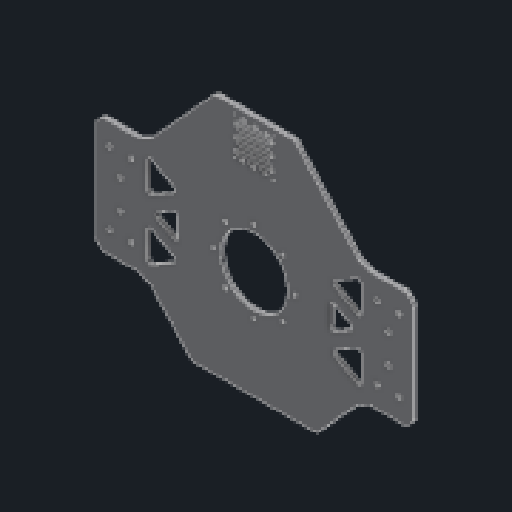
# Autodesk Inventor part: Root
Saved by Autodesk Inventor 2025.2 (Build 292293000, 293)
## iProperties
Created: 2020-05-07
Part Number: Root
Material: Generic
Document SubType Name: Sheet Metal
Designer: valer
Density: 1 g/cm^3
Sheet Metal Rule: Default
Appearance: Default
Author: valer
Autodesk Inventor part; units mm, degrees
ref_plane "YZ Plane" through (0, 0, 0) normal (1, 0, 0) x (0, 1, 0)
ref_plane "XZ Plane" through (0, 0, 0) normal (0, 1, 0) x (-1, 0, 0)
ref_plane "XY Plane" through (0, 0, 0) normal (0, 0, 1) x (1, 0, 0)
sketch "Base" plane through (0, 0, 0) normal (0, 0, 1) x (1, 0, 0)
  circle A0 centre (-56.25, 0) radius 2.75 construction
  circle A1 centre (0, -56.25) radius 2.75 construction
  circle A2 centre (0, 56.25) radius 2.75 construction
  circle A3 centre (39.7748, -39.7748) radius 2.75 construction
  circle A4 centre (-39.7748, 39.7748) radius 2.75 construction
  circle A5 centre (-39.7748, -39.7748) radius 2.75 construction
  circle A6 centre (39.7748, 39.7748) radius 2.75 construction
  circle A7 centre (56.25, 0) radius 2.75 construction
  circle A8 centre (0, 0) radius 45 construction
  circle A9 centre (0, 0) radius 61
  line L0 (220, 80) -> (-220, 80) construction
  line L1 (0, -210) -> (0, 210) construction
  line L2 (-308, 0) -> (308, 0) construction
  line L3 (-220, 80) -> (-150, 80)
  line L4 (-150, 80) -> (-150, 0)
  line L5 (-150, 0) -> (-220, 0)
  line L6 (-220, 0) -> (-220, 80)
  line L7 (86.6025, -150) -> (-86.6025, -150)
  line L8 (-86.6025, -150) -> (-173.2051, 0)
  line L9 (-173.2051, 0) -> (-86.6025, 150)
  line L10 (-86.6025, 150) -> (86.6025, 150)
  line L11 (86.6025, 150) -> (173.2051, 0)
  line L12 (173.2051, 0) -> (86.6025, -150)
  line L13 (-150, 0) -> (-86.6025, 150) construction
  line L14 (220, 80) -> (150, 80)
  line L15 (150, 80) -> (150, 0)
  line L16 (150, 0) -> (220, 0)
  line L17 (220, 0) -> (220, 80)
  line L18 (150, 0) -> (86.6025, 150) construction
  line L19 (-220, -80) -> (-150, -80)
  line L20 (-150, -80) -> (-150, 0)
  line L21 (-150, 0) -> (-219.7895, 0)
  line L22 (-219.7895, 0) -> (-220, -80)
  line L23 (-150, 0) -> (-86.6025, -150) construction
  line L24 (220, 0) -> (220, -80)
  line L25 (220, -80) -> (150, -80)
  line L26 (150, -80) -> (150, 0)
  line L27 (150, 0) -> (220, 0)
  line L28 (150, 0) -> (86.6025, -150) construction
  circle A10 centre (0, 0) radius 46.5
  circle A11 centre (-56.25, 0) radius 2.25
  circle A12 centre (-39.7748, -39.7748) radius 2.25
  circle A13 centre (0, -56.25) radius 2.25
  circle A14 centre (39.7748, -39.7748) radius 2.25
  circle A15 centre (56.25, 0) radius 2.25
  circle A16 centre (39.7748, 39.7748) radius 2.25
  circle A17 centre (0, 56.25) radius 2.25
  circle A18 centre (-39.7748, 39.7748) radius 2.25
  line L29 (-150, 80) -> (-86.6025, 150)
  line L30 (86.6025, 150) -> (150, 80)
  line L31 (-150, -80) -> (-86.6025, -150)
  line L32 (86.6025, -150) -> (150, -80)
  point P0 (0, 0)
  point P1 (210, 0)
  point P2 (150, 40.1924)
  point P3 (150, -40.1924)
  point P4 (173.2051, 0)
  point P5 (173.2051, 0)
  point P6 (-150, 40.1924)
  point P7 (-173.2051, 0)
  point P8 (-173.2051, 0)
  point P9 (-150, -40.1924)
  point P10 (173.2051, 0)
  point P11 (-173.2051, 0)
  point P12 (-173.2051, 0)
  dimension "d89" = 80
  dimension "d90" = 70
  dimension "d91" = 1.5
  dimension "d92" = 4.5
  dimension "d157" = 150
  dimension "d158" = 220
  measures "d89" distance between parallel lines of L0 L5
  measures "d90" distance between parallel lines of L4 L6
  measures "d91" radial gap between concentric circles of A10 A8
  measures "d92" diameter of A11
  measures "d157" distance from line of L7 A8.centre
  measures "d158" distance between parallel lines of L24 L1
extrude "Plate1" add sketch "Base" against normal blind 5 contours A9 | L3 L4 L9 L5 L6 | L29 L9 L4 | L9 L10 L11 L15 L26 L12 L7 L8 L20 L4 | L4 L5 L9 | L5 L8 L20 L19 L22 | L20 L8 L5 | L30 L15 L11 | L8 L31 L20 | L15 L14 L17 L16 L11 | L11 L16 L15 | L16 L24 L25 L26 L12 | L12 L26 L16 | L12 L26 L32
sketch "LegMountHoles" plane through (0, 0, -5) normal (0, 0, -1) x (-1, 0, 0)
  line L0 (-222.4542, 0) -> (-220, 0) construction
  line L1 (-220, 80) -> (-150, 80) construction
  line L2 (-185, 80) -> (-185, 0) construction
  line L3 (-170, 58) -> (-200, 58) construction
  circle A0 centre (-170, 58) radius 3
  circle A1 centre (-200, 58) radius 3
  circle A2 centre (-185, 18) radius 3
  line L4 (308.4908, 0) -> (-310.9451, 0) construction
  line L5 (0, -210) -> (0, 210) construction
  circle A3 centre (170, 58) radius 3
  circle A4 centre (200, 58) radius 3
  circle A5 centre (185, 18) radius 3
  circle A6 centre (-170, -58) radius 3
  circle A7 centre (-200, -58) radius 3
  circle A8 centre (-185, -18) radius 3
  circle A9 centre (170, -58) radius 3
  circle A10 centre (200, -58) radius 3
  circle A11 centre (185, -18) radius 3
  line L6 (-150, 80) -> (-86.6025, 150) projected
  line L7 (-220, -80) -> (-220, 80) projected
  point P0 (0, 0)
  point P1 (-185, 58)
  dimension "d93" = 6
  dimension "d94" = 30
  dimension "d95" = 40
  dimension "d161" = 18
  constraints: 12 centre point, 9 symmetric about line, 6 end point, 4 point on line, 2 coincident, 2 equal radius, 2 horizontal, 2 midpoint, 2 perpendicular, 1 collinear, 9 other
  measures "d93" diameter of A0
  measures "d94" distance of L3.start L3.end
  measures "d95" distance from line of L3 A2.centre
  measures "d161" distance from line of L4 A2.centre
extrude "LegMountHolesFeature" cut sketch "LegMountHoles" against normal blind 5
chamfer "OutsideChamfersFeature" distance 10 angle 45 8 edges at (-220, -80, -2.5) (-150, -80, -2.5) (150, -80, -2.5) (220, -80, -2.5) (-220, 80, -2.5) (-150, 80, -2.5) (150, 80, -2.5) (220, 80, -2.5)
fillet "OutsideFilletsFeature" radius 8 18 edges at (160, 80, -2.5) (210, 80, -2.5) (220, 70, -2.5) (210, -80, -2.5) (160, -80, -2.5) (86.6025, -150, -2.5) (-86.6025, -150, -2.5) (-160, -80, -2.5) (-210, -80, -2.5) (-219.9737, -70, -2.5) (-220, 0, -2.5) (-220, 70, -2.5) (-210, 80, -2.5) (-160, 80, -2.5) (-143.2871, 87.412, -2.5) (143.2871, 87.412, -2.5) (143.2871, -87.412, -2.5) (-143.2871, -87.412, -2.5)
sketch "LaserMount" plane through (0, 0, -5) normal (0, 0, -1) x (-1, 0, 0)
  line L0 (86.6025, 150) -> (142.1497, 88.6679)
  line L1 (86.6025, 150) -> (54.9038, 185)
  line L2 (54.9038, 185) -> (0, 185)
  line L3 (0, -217) -> (0, 252) construction
  line L4 (-86.6025, 150) -> (86.6025, 150)
  line L5 (-86.6025, 150) -> (-54.9038, 185)
  line L6 (-54.9038, 185) -> (0, 185)
  line L7 (86.6025, 150) -> (142.1497, 88.6679)
  point P0 (0, 0)
  dimension "d119" = 35
  measures "d119" distance between parallel lines of L2 L4
sheet face with bend "LaserMountFeature" sketch "LaserMount" thickness 5 toward (0, 0, 1) bend radius 5 relief straight relief width 5 relief depth 2.5
bend "Bend4"
fillet "FrontFilletsFeature" radius 8 2 edges at (-54.9038, 185, -2.5) (54.9038, 185, -2.5)
sketch "Sketch13" plane through (0, 0, -5) normal (0, 0, -1) x (-1, 0, 0)
  circle A0 centre (26.5, 175.5) radius 1
  circle A1 centre (26.5, 122.5) radius 1
  circle A2 centre (-26.5, 122.5) radius 1
  circle A3 centre (-26.5, 175.5) radius 1
  circle A4 centre (-26.5, 175.5) radius 1.5
  circle A5 centre (-26.5, 122.5) radius 1.5 construction
  arc A6 (26, 119.25) -> (29.75, 123) centre (26, 123) ccw construction
  line L0 (26, 119.25) -> (-26, 119.25) construction
  arc A7 (-29.75, 123) -> (-26, 119.25) centre (-26, 123) ccw construction
  line L1 (-29.75, 123) -> (-29.75, 175) construction
  arc A8 (-26, 178.75) -> (-29.75, 175) centre (-26, 175) ccw construction
  line L2 (-26, 178.75) -> (26, 178.75) construction
  arc A9 (29.75, 175) -> (26, 178.75) centre (26, 175) ccw construction
  line L3 (29.75, 175) -> (29.75, 123) construction
  circle A10 centre (26.5, 122.5) radius 1.5 construction
  circle A11 centre (-26.5, 175.5) radius 1.5 construction
  circle A12 centre (26.5, 175.5) radius 1.5
  circle A13 centre (-26.5, 122.5) radius 1.5 construction
  spline S0 degree 3 poles (23.6196, 120.808) (23.6757, 120.7125) (23.7146, 120.6074) (23.7573, 120.3902) (23.7611, 120.278) (23.7347, 120.0723) (23.7049, 119.9435) (23.5614, 119.6936) (23.4754, 119.5942) (23.2857, 119.4454) (23.1885, 119.3933) (22.9792, 119.3212) (22.8686, 119.3024) (22.7579, 119.3024) knots 0 0 0 0 0.207802 0.207802 0.415412 0.415412 0.597058 0.597058 0.743635 0.743635 0.871765 0.871765 1 1 1 1 construction
  arc A14 (28.192, 125.3804) -> (23.6196, 120.808) centre (26.5, 122.5) ccw construction
  spline S1 degree 3 poles (29.6976, 126.2421) (29.6976, 126.1314) (29.6779, 126.0211) (29.6047, 125.8121) (29.5512, 125.7135) (29.4244, 125.5497) (29.3335, 125.4537) (29.083, 125.3108) (28.9586, 125.2686) (28.7195, 125.2364) (28.6093, 125.2407) (28.3924, 125.2846) (28.2875, 125.3243) (28.192, 125.3804) knots 0 0 0 0 0.208148 0.208148 0.416054 0.416054 0.597577 0.597577 0.743842 0.743842 0.871851 0.871851 1 1 1 1 construction
  line L4 (29.6976, 171.7579) -> (29.6976, 126.2421) construction
  spline S2 degree 3 poles (28.192, 172.6196) (28.2875, 172.6757) (28.3926, 172.7146) (28.6098, 172.7573) (28.722, 172.7611) (28.9277, 172.7347) (29.0565, 172.7049) (29.3064, 172.5614) (29.4058, 172.4754) (29.5546, 172.2857) (29.6067, 172.1885) (29.6788, 171.9792) (29.6976, 171.8686) (29.6976, 171.7579) knots 0 0 0 0 0.207802 0.207802 0.415412 0.415412 0.597058 0.597058 0.743635 0.743635 0.871765 0.871765 1 1 1 1 construction
  arc A15 (23.6196, 177.192) -> (28.192, 172.6196) centre (26.5, 175.5) ccw construction
  spline S3 degree 3 poles (22.7579, 178.6976) (22.8686, 178.6976) (22.9789, 178.6779) (23.1879, 178.6047) (23.2865, 178.5512) (23.4503, 178.4244) (23.5463, 178.3335) (23.6892, 178.083) (23.7314, 177.9586) (23.7636, 177.7195) (23.7593, 177.6093) (23.7154, 177.3924) (23.6757, 177.2875) (23.6196, 177.192) knots 0 0 0 0 0.208148 0.208148 0.416054 0.416054 0.597577 0.597577 0.743842 0.743842 0.871851 0.871851 1 1 1 1 construction
  line L5 (-22.7579, 178.6976) -> (22.7579, 178.6976) construction
  spline S4 degree 3 poles (-23.6196, 177.192) (-23.6757, 177.2875) (-23.7146, 177.3926) (-23.7573, 177.6098) (-23.7611, 177.722) (-23.7347, 177.9277) (-23.7049, 178.0565) (-23.5614, 178.3064) (-23.4754, 178.4058) (-23.2857, 178.5546) (-23.1885, 178.6067) (-22.9792, 178.6788) (-22.8686, 178.6976) (-22.7579, 178.6976) knots 0 0 0 0 0.207802 0.207802 0.415412 0.415412 0.597058 0.597058 0.743635 0.743635 0.871765 0.871765 1 1 1 1 construction
  arc A16 (-28.192, 172.6196) -> (-23.6196, 177.192) centre (-26.5, 175.5) ccw construction
  spline S5 degree 3 poles (-29.6976, 171.7579) (-29.6976, 171.8686) (-29.6779, 171.9789) (-29.6047, 172.1879) (-29.5512, 172.2865) (-29.4244, 172.4503) (-29.3335, 172.5463) (-29.083, 172.6892) (-28.9586, 172.7314) (-28.7195, 172.7636) (-28.6093, 172.7593) (-28.3924, 172.7154) (-28.2875, 172.6757) (-28.192, 172.6196) knots 0 0 0 0 0.208148 0.208148 0.416054 0.416054 0.597577 0.597577 0.743842 0.743842 0.871851 0.871851 1 1 1 1 construction
  line L6 (-29.6976, 126.2421) -> (-29.6976, 171.7579) construction
  spline S6 degree 3 poles (-28.192, 125.3804) (-28.2875, 125.3243) (-28.3926, 125.2854) (-28.6098, 125.2427) (-28.722, 125.2389) (-28.9277, 125.2653) (-29.0565, 125.2951) (-29.3064, 125.4386) (-29.4058, 125.5246) (-29.5546, 125.7143) (-29.6067, 125.8115) (-29.6788, 126.0208) (-29.6976, 126.1314) (-29.6976, 126.2421) knots 0 0 0 0 0.207802 0.207802 0.415412 0.415412 0.597058 0.597058 0.743635 0.743635 0.871765 0.871765 1 1 1 1 construction
  arc A17 (-23.6196, 120.808) -> (-28.192, 125.3804) centre (-26.5, 122.5) ccw construction
  spline S7 degree 3 poles (-22.7579, 119.3024) (-22.8686, 119.3024) (-22.9789, 119.3221) (-23.1879, 119.3953) (-23.2865, 119.4488) (-23.4503, 119.5756) (-23.5463, 119.6665) (-23.6892, 119.917) (-23.7314, 120.0414) (-23.7636, 120.2805) (-23.7593, 120.3907) (-23.7154, 120.6076) (-23.6757, 120.7125) (-23.6196, 120.808) knots 0 0 0 0 0.208148 0.208148 0.416054 0.416054 0.597577 0.597577 0.743842 0.743842 0.871851 0.871851 1 1 1 1 construction
  line L7 (22.7579, 119.3024) -> (-22.7579, 119.3024) construction
  point P0 (0, 0)
  dimension "d130" = 2
  dimension "d131" = 2
  dimension "d132" = 2
  dimension "d133" = 2
  constraints: 4 centre point, 4 coincident
  measures "d130" diameter of A0
  measures "d131" diameter of A1
  measures "d132" diameter of A2
  measures "d133" diameter of A3
extrude "LaserMountHolesFeature" cut sketch "Sketch13" against normal blind 5 contours A0 | A1 | A2 | A3
sketch "LaserVentHoles" plane through (0, 0, -5) normal (0, 0, -1) x (-1, 0, 0)
  line L0 (23.5, 148.3368) -> (0.6632, 125.5) construction
  line L1 (21.3787, 150.4581) -> (-1.4581, 127.6213)
  line L2 (2.7846, 123.3787) -> (25.6213, 146.2154)
  arc A0 (25.6213, 146.2154) -> (21.3787, 150.4581) centre (23.5, 148.3368) ccw
  arc A1 (-1.4581, 127.6213) -> (2.7846, 123.3787) centre (0.6632, 125.5) ccw
  line L3 (16.7721, 125.5) -> (23.5, 132.2279) construction
  line L4 (18.8934, 123.3787) -> (25.6213, 130.1066)
  line L5 (21.3787, 134.3492) -> (14.6508, 127.6213)
  arc A2 (14.6508, 127.6213) -> (18.8934, 123.3787) centre (16.7721, 125.5) ccw
  arc A3 (25.6213, 130.1066) -> (21.3787, 134.3492) centre (23.5, 132.2279) ccw
  line L6 (0, -217) -> (0, 252) construction
  circle A4 centre (26.5, 122.5) radius 1 projected
  circle A5 centre (26.5, 175.5) radius 1 projected
  circle A6 centre (-26.5, 175.5) radius 1 projected
  circle A7 centre (-26.5, 122.5) radius 1 projected
  line L7 (26.5, 122.5) -> (-26.5, 122.5) construction
  line L8 (-26.5, 122.5) -> (-26.5, 175.5) construction
  line L9 (-26.5, 175.5) -> (26.5, 175.5) construction
  line L10 (26.5, 175.5) -> (26.5, 122.5) construction
  line L11 (23.5, 164.4456) -> (-15.4456, 125.5) construction
  line L12 (21.3787, 166.5669) -> (-17.5669, 127.6213)
  line L13 (-13.3243, 123.3787) -> (25.6213, 162.3243)
  arc A8 (25.6213, 162.3243) -> (21.3787, 166.5669) centre (23.5, 164.4456) ccw
  arc A9 (-17.5669, 127.6213) -> (-13.3243, 123.3787) centre (-15.4456, 125.5) ccw
  line L14 (15.4456, 172.5) -> (-23.5, 133.5544) construction
  line L15 (17.5669, 170.3787) -> (-21.3787, 131.4331)
  line L16 (-25.6213, 135.6757) -> (13.3243, 174.6213)
  arc A10 (17.5669, 170.3787) -> (13.3243, 174.6213) centre (15.4456, 172.5) ccw
  arc A11 (-25.6213, 135.6757) -> (-21.3787, 131.4331) centre (-23.5, 133.5544) ccw
  line L17 (-0.6632, 172.5) -> (-23.5, 149.6632) construction
  line L18 (-2.7846, 174.6213) -> (-25.6213, 151.7846)
  line L19 (-21.3787, 147.5419) -> (1.4581, 170.3787)
  arc A12 (1.4581, 170.3787) -> (-2.7846, 174.6213) centre (-0.6632, 172.5) ccw
  arc A13 (-25.6213, 151.7846) -> (-21.3787, 147.5419) centre (-23.5, 149.6632) ccw
  line L20 (-16.7721, 172.5) -> (-23.5, 165.7721) construction
  line L21 (-18.8934, 174.6213) -> (-25.6213, 167.8934)
  line L22 (-21.3787, 163.6508) -> (-14.6508, 170.3787)
  arc A14 (-14.6508, 170.3787) -> (-18.8934, 174.6213) centre (-16.7721, 172.5) ccw
  arc A15 (-25.6213, 167.8934) -> (-21.3787, 163.6508) centre (-23.5, 165.7721) ccw
  point P0 (0, 0)
  point P1 (12.0816, 136.9184)
  point P2 (20.136, 128.864)
  point P3 (4.0272, 144.9728)
  point P4 (-4.0272, 153.0272)
  point P5 (-12.0816, 161.0816)
  point P6 (-20.136, 169.136)
  dimension "d136" = 45
  dimension "d137" = 3
  dimension "d138" = 6
  dimension "d139" = 11.3907
  dimension "d140" = 11.3907
  dimension "d141" = 11.3907
  dimension "d142" = 11.3907
  dimension "d143" = 11.3907
  constraints: 56 end point, 36 tangent, 24 point on circle, 15 parallel, 12 centre point, 6 midpoint, 5 equal radius, 1 horizontal, 1 perpendicular
  measures "d136" angle of L6 L3
  measures "d137" radius of A2
  measures "d138" distance from line of L4 L7.start
  measures "d139" distance between parallel lines of L0 L3
  measures "d140" distance between parallel lines of L11 L0
  measures "d141" distance between parallel lines of L14 L11
  measures "d142" distance between parallel lines of L17 L14
  measures "d143" distance between parallel lines of L20 L17
extrude "LaserVentHolesFeature" cut sketch "LaserVentHoles" against normal blind 5 contours A0 L2 A1 L1 | A2 L5 A3 L4 | A8 L13 A9 L12 | L15 A11 L16 A10 | A12 L19 A13 L18 | A14 L22 A15 L21
sketch "TrianglePattern" plane through (0, 0, -5) normal (0, 0, -1) x (-1, 0, 0)
  line L0 (-148.3013, -66.7074) -> (-105, -41.7074)
  line L1 (-105, -41.7074) -> (-148.3013, -16.7074)
  line L2 (-148.3013, -16.7074) -> (-148.3013, -66.7074)
  line L3 (-139.641, 0) -> (-105, -20)
  line L4 (-105, -20) -> (-105, 20)
  line L5 (-105, 20) -> (-139.641, 0)
  line L6 (308, 0) -> (-308, 0) construction
  line L7 (-148.3013, 66.7074) -> (-105, 41.7074)
  line L8 (-105, 41.7074) -> (-148.3013, 16.7074)
  line L9 (-148.3013, 16.7074) -> (-148.3013, 66.7074)
  line L10 (0, -217) -> (0, 252) construction
  line L11 (148.3013, -66.7074) -> (105, -41.7074)
  line L12 (105, -41.7074) -> (148.3013, -16.7074)
  line L13 (148.3013, -16.7074) -> (148.3013, -66.7074)
  line L14 (139.641, 0) -> (105, -20)
  line L15 (105, -20) -> (105, 20)
  line L16 (105, 20) -> (139.641, 0)
  line L17 (148.3013, 16.7074) -> (148.3013, 66.7074)
  line L18 (148.3013, 66.7074) -> (105, 41.7074)
  line L19 (105, 41.7074) -> (148.3013, 16.7074)
  line L20 (-105, 41.7074) -> (-105, 20) construction
  line L21 (-105, 41.7074) -> (-148.3013, 41.7074) construction
  line L22 (-105, -41.7074) -> (-148.3013, -41.7074) construction
  point P0 (0, 0)
  dimension "d149" = 30
  dimension "d150" = 18.7992
  dimension "d151" = 30
  dimension "d152" = 30
  dimension "d153" = 18.7992
  dimension "d154" = 40
  dimension "d155" = 50
  dimension "d156" = 105
  constraints: 42 end point, 12 symmetric about line, 4 parallel, 2 midpoint, 1 collinear, 1 perpendicular, 1 point on line
  measures "d149" angle of L6 L5
  measures "d150" distance between parallel lines of L5 L8
  measures "d151" angle of L8 L21
  measures "d152" angle of L22 L1
  measures "d153" distance between parallel lines of L1 L3
  measures "d154" distance of L3.end L4.end
  measures "d155" distance of L9.start L9.end
  measures "d156" distance from line of L4 point (0, 0)
extrude "TriangleHolesFeature" cut sketch "TrianglePattern" against normal blind 5
fillet "TriangleHoleFilletsFeature" radius 4 18 edges at (105, -20, -2.5) (105, 20, -2.5) (139.641, 0, -2.5) (105, -41.7074, -2.5) (148.3013, -16.7074, -2.5) (148.3013, -66.7074, -2.5) (105, 41.7074, -2.5) (148.3013, 66.7074, -2.5) (148.3013, 16.7074, -2.5) (-148.3013, 66.7074, -2.5) (-148.3013, 16.7074, -2.5) (-105, 41.7074, -2.5) (-139.641, 0, -2.5) (-105, 20, -2.5) (-105, -20, -2.5) (-148.3013, -16.7074, -2.5) (-148.3013, -66.7074, -2.5) (-105, -41.7074, -2.5)
equation "\"d97\" = Thickness"
equation "\"d33\" = Thickness"
equation "\"BendRadius\" = Thickness"
equation "\"BendReliefWidth\" = Thickness"
equation "\"BendReliefDepth\" = 0.5 * Thickness"
equation "\"TransitionRadius\" = BendRadius"
equation "\"JacobiRadiusSize\" = BendRadius"
equation "\"GapSize\" = Thickness"
equation "\"Thickness\" = 5"
body "Solid1"
